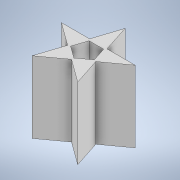
# Autodesk Inventor part: Star
Saved by Autodesk Inventor 2020.3 (Build 243373000, 373)
## iProperties
Created: 2021-05-21
Part Number: Star
Material: Generic
Document SubType Name: Modeling
Designer: patry
Density: 1 g/cm^3
Appearance: Default
Author: patry
Autodesk Inventor part; units mm, degrees
ref_plane "YZ Plane" through (0, 0, 0) normal (1, 0, 0) x (0, 1, 0)
ref_plane "XZ Plane" through (0, 0, 0) normal (0, 1, 0) x (-1, 0, 0)
ref_plane "XY Plane" through (0, 0, 0) normal (0, 0, 1) x (1, 0, 0)
sketch "Sketch1" plane through (0, 0, 0) normal (0, 1, 0) x (-1, 0, 0)
  line L0 (0, 0) -> (0, 14)
  line L1 (10.1716, 14) -> (16.458, -5.3475)
  line L2 (16.458, -5.3475) -> (0, -17.305)
  line L3 (0, -17.305) -> (-16.458, -5.3475)
  line L4 (-16.458, -5.3475) -> (-10.1716, 14)
  line L5 (-10.1716, 14) -> (10.1716, 14)
  line L6 (0, -17.305) -> (10.1716, 14)
  line L7 (-10.1716, 14) -> (0, -17.305)
  line L8 (16.458, -5.3475) -> (-16.458, -5.3475)
  line L9 (-16.458, -5.3475) -> (10.1716, 14)
  line L10 (16.458, -5.3475) -> (-10.1716, 14)
  line L11 (0, 0) -> (0, -4.5)
  line L12 (-3.2694, -4.5) -> (-5.2901, 1.7188)
  line L13 (-5.2901, 1.7188) -> (0, 5.5623)
  line L14 (0, 5.5623) -> (5.2901, 1.7188)
  line L15 (5.2901, 1.7188) -> (3.2694, -4.5)
  line L16 (3.2694, -4.5) -> (-3.2694, -4.5)
  point P0 (-3.8852, -5.3475)
  point P1 (3.8852, -5.3475)
  point P2 (6.2864, 2.0426)
  point P3 (0, 6.6099)
  point P4 (-6.2864, 2.0426)
  dimension "d0" = 14
  dimension "d3" = 4.5
  constraints: 34 end point, 2 coincident, 2 midpoint, 2 vertical, 1 horizontal, 22 other
  measures "d0" distance of L0.start L0.end
  measures "d3" distance of L11.start L11.end
extrude "Extrusion2" add sketch "Sketch1" along normal blind 32 contours L10 L6 L8 L7 L9 | L9 L7 L10 | L9 L6 L10 | L7 L8 L9 | L10 L8 L6 | L8 L6 L7
body "Solid2"
